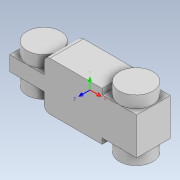
# Autodesk Inventor part: body
Saved by Autodesk Inventor 2020 (Build 240168000, 168)
## iProperties
Created: 2021-01-29
Part Number: body
Material: Generic
Document SubType Name: Modeling
Designer: DELL
Density: 1 g/cm^3
Appearance: Default
Author: DELL
Autodesk Inventor part; units mm, degrees
ref_plane "YZ Plane" through (0, 0, 0) normal (1, 0, 0) x (0, 1, 0)
ref_plane "XZ Plane" through (0, 0, 0) normal (0, 1, 0) x (-1, 0, 0)
ref_plane "XY Plane" through (0, 0, 0) normal (0, 0, 1) x (1, 0, 0)
sketch "Sketch1" plane through (0, 0, 0) normal (0, 0, 1) x (1, 0, 0)
  line L0 (-170, 20) -> (-77.5, 20)
  line L1 (170, 45) -> (170, 35)
  line L2 (-77.5, -20) -> (-170, -20)
  line L3 (-170, -20) -> (-170, 20)
  line L4 (-77.5, 65) -> (77.5, 65)
  line L5 (77.5, -65) -> (-77.5, -65)
  line L6 (170, 50) -> (77.5, 50)
  line L7 (77.5, -50) -> (170, -50)
  line L8 (170, -50) -> (170, 50)
  line L9 (-77.5, -65) -> (-77.5, -20)
  line L10 (-77.5, 20) -> (-77.5, 65)
  line L11 (-77.5, -20) -> (-77.5, -63.8623)
  line L12 (-170, 0) -> (170, 0) construction
  line L13 (77.5, -50) -> (77.5, -65)
  line L14 (77.5, 65) -> (77.5, 50)
  line L15 (62.5, 35) -> (155, 35)
  line L16 (155, 35) -> (155, -35)
  line L17 (155, -35) -> (62.5, -35)
  line L18 (62.5, -35) -> (62.5, -50)
  line L19 (62.5, -50) -> (-62.5, -50)
  line L20 (-62.5, -50) -> (-62.5, -5)
  line L21 (-62.5, -5) -> (-62.5, 50)
  line L22 (-62.5, 50) -> (62.5, 50)
  line L23 (62.5, 50) -> (62.5, 35)
  line L24 (0, 50) -> (0, -50) construction
  point P0 (0, 0)
  point P1 (170, 5)
  point P2 (170, -5)
  dimension "d2" = 155
  dimension "d3" = 130
  dimension "d21" = 92.5
  dimension "d22" = 100
  dimension "d23" = 40
  dimension "d25" = 92.5
  dimension "d29" = 15
  constraints: 50 end point, 7 collinear, 6 midpoint, 6 parallel, 4 horizontal, 1 perpendicular, 1 point on line, 1 vertical, 9 other
  measures "d2" distance of L4.start L4.end
  measures "d3" distance between parallel lines of L4 L5
  measures "d21" distance of L6.start L6.end
  measures "d22" distance between parallel lines of L6 L7
  measures "d23" distance between parallel lines of L0 L2
  measures "d25" distance between parallel lines of L10 L3
  measures "d29" distance between parallel lines of L6 L15
extrude "Extrusion1" add sketch "Sketch1" along normal mid plane 90 contours L0 L10 L4 L14 L6 L8 L1 L7 L13 L5 L9 L2 L3 | L15 L16 L17 L18 L19 L20 L21 L22 L23
sketch "Sketch2" plane through (0, 0, 0) normal (0, 1, 0) x (-1, 0, 0)
  circle A0 centre (-123.75, 0) radius 45
  circle A1 centre (123.75, 0) radius 45
  line L0 (0, 43.1567) -> (0, -43.1567) construction
  line L1 (170.8168, 0) -> (-169.1832, 0) construction
  line L2 (170.8168, 0) -> (-169.1832, 0) construction
  line L3 (170, -45) -> (170, 45) construction
  line L4 (77.5, -45) -> (170, -45) construction
  line L5 (123.75, -45) -> (123.75, 45) construction
  line L6 (170, 45) -> (77.5, 45) construction
  line L7 (-123.75, -45) -> (-123.75, 45) construction
  point P0 (0, 0)
  point P1 (0.8168, 0)
  point P2 (0, 0)
  dimension "d7" = 90
  constraints: 10 end point, 6 midpoint, 4 point on line, 2 centre point, 1 equal radius, 1 horizontal, 1 horizontal alignment, 1 symmetric about line, 1 other
  measures "d7" diameter of A0
extrude "Extrusion2" add sketch "Sketch2" against normal blind 32 from surface at -50 contours A0
extrude "Extrusion3" add sketch "Sketch2" against normal blind 32 from surface at -20 contours A1
fillet "Fillet1" radius 15 2 edges at (-77.5, 65, 0) (-77.5, -65, 0)
mirror "Mirror1" about plane through (0, 0, 0) normal (0, 1, 0) of "Extrusion3", "Extrusion2"
extrude "Extrusion4" cut sketch "Sketch1" against normal mid plane 55 contours L15 L16 L17 L18 L19 L20 L21 L22 L23
body "Solid1"
